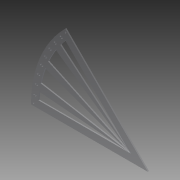
# Autodesk Inventor part: Side Panel
Saved by Autodesk Inventor 2013 (Build 170138000, 138)
## iProperties
Created: 2013-01-27
Part Number: Side Panel
Material: Polycarbonate, Clear
Document SubType Name: Modeling
Designer: Andrew Toennies
Density: 1.2 g/cm^3
Mass: 86.4397 g
Surface Area: 528.255 cm^2
Volume: 72.0331 cm^3
Author: Andrew Toennies
Autodesk Inventor part; units mm, degrees
ref_plane "YZ Plane" through (0, 0, 0) normal (1, 0, 0) x (0, 1, 0)
ref_plane "XZ Plane" through (0, 0, 0) normal (0, 1, 0) x (-1, 0, 0)
ref_plane "XY Plane" through (0, 0, 0) normal (0, 0, 1) x (1, 0, 0)
sketch "Sketch1" plane through (0, 0, 0) normal (0, 0, 1) x (1, 0, 0)
  arc A0 (-220.016275, 220.016275) -> (-311.15, 0) centre (0, 0) ccw
  line L0 (-311.15, 0) -> (-304.8, 0)
  line L1 (0, 0) -> (-220.016275, 220.016275)
  line L2 (-311.15, 0) -> (0, 0)
  constraints: 6 end point, 2 point on circle, 1 centre point
extrude "Extrusion1" add sketch "Sketch1" along normal blind 3.175
sketch "Sketch4" plane through (0, 0, 0) normal (0, 0, -1) x (-1, 0, 0)
  arc A0 (311.15, 0) -> (220.016275, 220.016275) centre (0, 0) ccw
  line L0 (220.016275, 220.016275) -> (0, 0)
  line L1 (0, 0) -> (311.15, 0)
  arc A1 (301.625, 0) -> (213.281083, 213.281083) centre (0, 0) ccw
  arc A2 (303.2125, 0) -> (214.403615, 214.403615) centre (0, 0) ccw
  arc A3 (304.8, 0) -> (215.526147, 215.526147) centre (0, 0) ccw construction
  arc A4 (300.0375, 0) -> (212.158551, 212.158551) centre (0, 0) ccw construction
  circle A5 centre (215.526147, 215.526147) radius 1.5875
  circle A6 centre (212.158551, 212.158551) radius 1.5875
  circle A7 centre (233.490346, 195.921663) radius 1.5875
  circle A8 centre (229.84206, 192.860387) radius 1.5875
  circle A9 centre (249.677543, 174.826098) radius 1.5875
  circle A10 centre (245.776331, 172.09444) radius 1.5875
  circle A11 centre (263.964543, 152.4) radius 1.5875
  circle A12 centre (259.840097, 150.01875) radius 1.5875
  circle A13 centre (276.242613, 128.814046) radius 1.5875
  circle A14 centre (271.926323, 126.801327) radius 1.5875
  circle A15 centre (286.418311, 104.24774) radius 1.5875
  circle A16 centre (281.943025, 102.618869) radius 1.5875
  circle A17 centre (294.414192, 78.888045) radius 1.5875
  circle A18 centre (289.81397, 77.655419) radius 1.5875
  circle A19 centre (300.169403, 52.927965) radius 1.5875
  circle A20 centre (295.479256, 52.100965) radius 1.5875
  circle A21 centre (303.640144, 26.56507) radius 1.5875
  circle A22 centre (298.895767, 26.149991) radius 1.5875
  circle A23 centre (304.8, 0) radius 1.5875
  circle A24 centre (300.0375, 0) radius 1.5875
  circle A25 centre (219.969498, 210.989242) radius 1.5875
  circle A26 centre (304.733847, 6.35) radius 1.5875
  point P0 (231.058155, 193.880813)
  point P1 (232.274251, 194.901238)
  point P2 (247.076735, 173.004993)
  point P3 (248.377139, 173.915545)
  point P4 (261.214912, 150.8125)
  point P5 (262.589728, 151.60625)
  point P6 (273.365086, 127.472233)
  point P7 (274.80385, 128.14314)
  point P8 (283.434787, 103.161826)
  point P9 (284.926549, 103.704783)
  point P10 (291.347377, 78.066294)
  point P11 (292.880785, 78.47717)
  point P12 (297.042639, 52.376632)
  point P13 (298.606021, 52.652298)
  point P14 (300.477226, 26.288351)
  point P15 (302.058685, 26.426711)
  point P16 (301.625, 0)
  point P17 (303.2125, 0)
  dimension "d2" = 9.525
  dimension "d3" = 1.5875
  dimension "d4" = 1.5875
  dimension "d5" = 1.5875
  dimension "d8" = 45
  dimension "d10" = 6.35
  dimension "d13" = 3.175
  dimension "d14" = 6.35
  constraints: 10 point on circle, 6 centre point, 2 coincident, 2 horizontal alignment, 2 point on line, 1 tangent, 113 other
  measures "d2" radial gap between concentric circles of A0 A1
  measures "d3" radial gap between concentric circles of A2 A1
  measures "d4" radial gap between concentric circles of A4 A1
  measures "d5" radial gap between concentric circles of A3 A2
  measures "d10" distance from line of L0 A25.centre
  measures "d13" diameter of A26
  measures "d14" distance from line of L1 A26.centre
sketch "Sketch4 outline for Extrusion2" plane through (0, 0, 0) normal (0, 0, -1) x (-1, 0, 0)
  circle A0 centre (233.490346, 195.921663) radius 1.5875
  circle A1 centre (249.677543, 174.826098) radius 1.5875
  circle A2 centre (263.964543, 152.4) radius 1.5875
  circle A3 centre (276.242613, 128.814046) radius 1.5875
  circle A4 centre (286.418311, 104.24774) radius 1.5875
  circle A5 centre (294.414192, 78.888045) radius 1.5875
  circle A6 centre (300.169403, 52.927965) radius 1.5875
  circle A7 centre (303.640144, 26.56507) radius 1.5875
  circle A8 centre (219.969498, 210.989242) radius 1.5875
  circle A9 centre (304.733847, 6.35) radius 1.5875
  circle A10 centre (229.84206, 192.860387) radius 1.5875
  circle A11 centre (245.776331, 172.09444) radius 1.5875
  circle A12 centre (259.840097, 150.01875) radius 1.5875
  circle A13 centre (271.926323, 126.801327) radius 1.5875
  circle A14 centre (281.943025, 102.618869) radius 1.5875
  circle A15 centre (289.81397, 77.655419) radius 1.5875
  circle A16 centre (295.479256, 52.100965) radius 1.5875
  circle A17 centre (298.895767, 26.149991) radius 1.5875
extrude "Extrusion2" cut sketch "Sketch4 outline for Extrusion2" against normal blind 25.4
sketch "Sketch7" plane through (0, 0, 3.175) normal (0, 0, 1) x (1, 0, 0)
  line L0 (-219.576555, 192.635787) -> (-45.990768, 19.05)
  line L1 (-45.990768, 19.05) -> (-291.478142, 19.05)
  arc A0 (-99.872305, 72.931537) -> (-122.190768, 19.05) centre (-45.990768, 19.05) ccw
  dimension "d29" = 152.4
  constraints: 2 point on circle, 2 point on line, 1 centre point, 1 coincident
  measures "d29" diameter of A0
extrude "Extrusion4" add sketch "Sketch7" against normal blind 3.175
sketch "Sketch9" plane through (0, 0, 3.175) normal (0, 0, 1) x (1, 0, 0)
  arc A0 (-220.016275, 220.016275) -> (-311.15, 0) centre (0, 0) ccw
  line L0 (0, 0) -> (-220.016275, 220.016275)
  arc A1 (-219.576555, 192.635787) -> (-291.478142, 19.05) centre (0, 0) ccw
  arc A2 (-201.574062, 174.633294) -> (-266.132217, 17.393478) centre (0, 0) ccw
  arc A3 (-181.389328, 159.133911) -> (-240.786292, 15.736957) centre (0, 0) ccw
  arc A4 (-162.295715, 142.382973) -> (-215.440366, 14.080435) centre (0, 0) ccw
  arc A5 (-143.202101, 125.632035) -> (-190.094441, 12.423913) centre (0, 0) ccw
  arc A6 (-124.108488, 108.881097) -> (-164.748515, 10.767391) centre (0, 0) ccw
  arc A7 (-105.014874, 92.130159) -> (-139.40259, 9.11087) centre (0, 0) ccw
  arc A8 (-66.827647, 58.628283) -> (-88.710739, 5.797826) centre (0, 0) ccw
  line L1 (-219.576555, 192.635787) -> (-201.574062, 174.633294)
  line L2 (-266.132217, 17.393478) -> (-291.478142, 19.05)
  line L3 (-215.440366, 14.080435) -> (-240.786292, 15.736957)
  line L4 (-88.710739, 5.797826) -> (-139.40259, 9.11087)
  line L5 (-164.748515, 10.767391) -> (-190.094441, 12.423913)
  line L6 (-66.827647, 58.628283) -> (-105.014874, 92.130159)
  line L7 (-143.202101, 125.632035) -> (-124.108488, 108.881097)
  line L8 (-181.389328, 159.133911) -> (-162.295715, 142.382973)
  dimension "d34" = 19.05
  dimension "d35" = 25.4
  dimension "d36" = 25.4
  dimension "d38" = 25.4
  dimension "d39" = 25.4
  dimension "d40" = 25.4
  dimension "d41" = 25.4
  constraints: 17 point on circle, 16 end point, 8 centre point, 2 collinear, 1 parallel
  measures "d34" radial gap between concentric circles of A0 A1
  measures "d35" radial gap between concentric circles of A1 A2
  measures "d36" radial gap between concentric circles of A2 A3
  measures "d38" radial gap between concentric circles of A4 A3
  measures "d39" radial gap between concentric circles of A5 A4
  measures "d40" radial gap between concentric circles of A5 A6
  measures "d41" radial gap between concentric circles of A6 A7
extrude "Extrusion5" cut sketch "Sketch9" against normal blind 3.175
body "Solid1"
